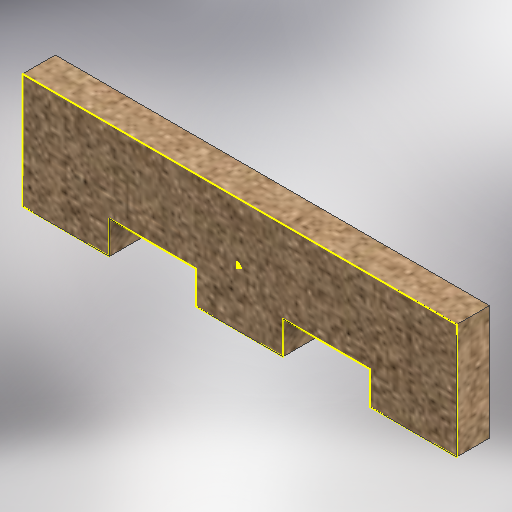
# Autodesk Inventor part: wall1
Saved by Autodesk Inventor 2025 (Build 290162000, 162)
## iProperties
Created: 2024-09-26
Part Number: wall1
Material: MDF Medium Density Fiberboard
Document SubType Name: Modeling
Designer: DANIEL
Density: 0.8 g/cm^3
Appearance: Cardboard - Corrugated
Checked By: FERNANDO
Engr Approved By: ANTONIO
Stock Number: 2
Author: DANIEL
Title: WALL 1
Autodesk Inventor part; units mm, degrees
ref_plane "YZ Plane" through (0, 0, 0) normal (1, 0, 0) x (0, 1, 0)
ref_plane "XZ Plane" through (0, 0, 0) normal (0, 1, 0) x (-1, 0, 0)
ref_plane "XY Plane" through (0, 0, 0) normal (0, 0, 1) x (1, 0, 0)
sketch "Sketch1" plane through (0, 0, 0) normal (0, 0, 1) x (1, 0, 0)
  line L0 (-26.5, 7) -> (26.5, 7)
  line L1 (26.5, 7) -> (26.5, -7)
  line L2 (26.5, -7) -> (-26.5, -7)
  line L3 (-26.5, -7) -> (-26.5, 7)
  line L4 (-26.5, 7) -> (26.5, -7) construction
  line L5 (26.5, 7) -> (-26.5, -7) construction
  line L6 (26.5, -7) -> (15.9, -7)
  line L7 (15.9, -7) -> (15.9, -3)
  line L8 (15.9, -3) -> (26.5, -3)
  line L9 (26.5, -3) -> (26.5, -7)
  line L10 (5.3, -7) -> (5.3, -3)
  line L11 (5.3, -3) -> (15.9, -3)
  line L12 (-5.3, -7) -> (-5.3, -3)
  line L13 (-5.3, -3) -> (5.3, -3)
  line L14 (-15.9, -7) -> (-15.9, -3)
  line L15 (-15.9, -3) -> (-5.3, -3)
  line L16 (-26.5, -7) -> (-26.5, -3)
  line L17 (-26.5, -3) -> (-15.9, -3)
  point P0 (0, 0)
  dimension "d0" = 53
  dimension "d1" = 14
  dimension "d2" = 10.6
  dimension "d3" = 4
  dimension "d6" = 10.6
  constraints: 36 end point, 4 parallel, 3 horizontal, 2 midpoint, 2 perpendicular, 20 other
  measures "d0" distance of L1.end L2.end
  measures "d1" distance of L0.end L1.end
  measures "d2" distance of L7.end L8.end
  measures "d3" distance of L6.end L7.end
  measures "d6" distance of L6.end L10.start
extrude "Extrusion1" add sketch "Sketch1" along normal blind 4 contours L0 L1 L8 L11 L13 L15 L17 L3 | L17 L14 L2 L3 | L1 L2 L7 L8 | L13 L10 L2 L12
sketch "Sketch2" plane through (0, 0, 4) normal (0, 0, 1) x (1, 0, 0)
  line L0 (-26.5, 7) -> (-26.5, -7) projected
  line L1 (-26.5, -7) -> (-15.9, -7) projected
  line L2 (-15.9, -7) -> (-15.9, -3) projected
  line L3 (-15.9, -3) -> (-5.3, -3) projected
  line L4 (-5.3, -3) -> (-5.3, -7) projected
  line L5 (-5.3, -7) -> (5.3, -7) projected
  line L6 (5.3, -7) -> (5.3, -3) projected
  line L7 (5.3, -3) -> (15.9, -3) projected
  line L8 (15.9, -3) -> (15.9, -7) projected
  line L9 (15.9, -7) -> (26.5, -7) projected
  line L10 (26.5, -7) -> (26.5, 7) projected
  line L11 (26.5, 7) -> (-26.5, 7) projected
  point P0 (0, 0)
equation "\"d1\" = height + e"
equation "\"d2\" = 0.2 * d0"
equation "\"d3\" = e"
equation "\"d6\" = d2"
equation "\"d11\" = e"
equation "\"e\" = 4"
equation "\"height\" = 10"
body "Solid1"
